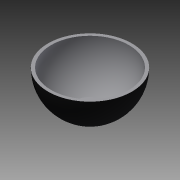
# Autodesk Inventor part: ORB-bottom
Saved by Autodesk Inventor 2015 (Build 190159000, 159)
## iProperties
Created: 2014-12-21
Part Number: ORB-bottom
Material: Generic
Document SubType Name: Modeling
Designer: Sudhar
Density: 1 g/cm^3
Appearance: Default
Author: Sudhar
Autodesk Inventor part; units mm, degrees
ref_plane "YZ Plane" through (0, 0, 0) normal (1, 0, 0) x (0, 1, 0)
ref_plane "XZ Plane" through (0, 0, 0) normal (0, 1, 0) x (-1, 0, 0)
sketch "Sketch1" plane through (0, 0, 0) normal (0, 0, 1) x (1, 0, 0)
  arc A0 (-4.0424, -42.6815) -> (40.4076, 1.7685) centre (-4.0424, 1.7685) ccw
  line L0 (-4.0424, 1.7685) -> (40.4076, 1.7685)
  line L1 (-4.0424, 1.7685) -> (-4.0424, -42.6815)
  dimension "d0" = 88.9
  constraints: 4 end point, 2 point on circle, 1 centre point, 1 vertical
  measures "d0" diameter of A0
revolve "Revolution1" add sketch "Sketch1" angle 360 about axis through (-4.0424, 1.7685, 0) along (0, -1, 0)
ref_plane "Work Plane2" through (-4.0424, 1.7685, 44.45) normal (0, 0, 1) x (1, 0, 0)
sketch "Sketch3" plane through (-4.0424, 1.7685, 44.45) normal (0, 0, 1) x (1, 0, 0)
  line L0 (-27.3232, -41.3412) -> (29.0699, -41.3412)
  constraints: 2 end point, 1 horizontal
surface extrude "ExtrusionSrf2" sketch "Sketch3" against normal blind 127 shown no curves L0
split body "Split2" result one side removed by surface "ExtrusionSrf2" removed pieces at (7.0948, -40.569, -3.8851)
shell "Shell2" thickness 3.175 removed faces 1 at (-16.0293, 1.7685, -8.709)
body "Solid1"
body "Srf2"
